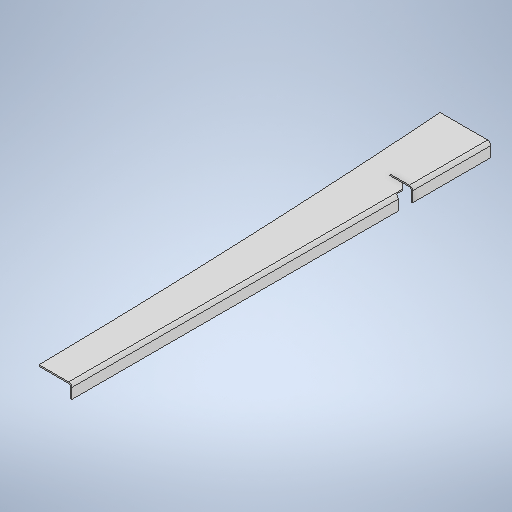
# Autodesk Inventor part: MSC 054 rib hip 1
Saved by Autodesk Inventor 2025 (Build 290162010, 162A)
## iProperties
Created: 2024-04-28
Part Number: MSC 054 rib hip 1
Material: Stainless Steel
Document SubType Name: Sheet Metal
Designer: pokla
Stock Number: МОО 054 шпангоут бедро 1
Density: 8 g/cm^3
Flat Pattern Width: 61.5 cm
Flat Pattern Length: 9.06945 cm
Flat Pattern Area: 557.771 cm^2
Sheet Metal Rule: AISI304 2mm Die16
Sheet Metal Width: 615,000 mm
Sheet Metal Length: 90,694 mm
Sheet Metal Area: 55777,098 mm^2
Appearance: Default
Стрингер_3: 66,766 mm
Стрингер_4: 48,009 mm
Стрингер_5: 51,895 mm
Стрингер_6: 78,448 mm
Author: admin
Autodesk Inventor part; units mm, degrees
ref_plane "YZ Plane" through (0, 0, 0) normal (1, 0, 0) x (0, 1, 0)
ref_plane "XZ Plane" through (0, 0, 0) normal (0, 1, 0) x (-1, 0, 0)
ref_plane "XY Plane" through (0, 0, 0) normal (0, 0, 1) x (1, 0, 0)
sketch "Sketch1" plane through (0, 0, 0) normal (0, 0, 1) x (1, 0, 0)
  arc A0 (750, -2100) -> (771.0671, -250.888) centre (-10250, -1050) ccw construction
  arc A1 (752.9864, -2100.2851) -> (772.2226, -225.7318) centre (-10246.9893, -1050.0309) ccw
  line L0 (-750, -2700) -> (-750, 0) construction
  line L1 (-800, 50) -> (-800, -2750) construction
  line L2 (-850, -2800) -> (-850, 100) construction
  line L3 (850, 100) -> (850, -2800)
  line L4 (800, -2750) -> (800, 50) construction
  line L5 (750, 0) -> (750, -2700) construction
  line L6 (771.0671, -250.888) -> (768.075, -251.105) construction
  line L7 (769.231, -225.9556) -> (772.2226, -225.7318) construction
  arc A2 (747.4657, -5.0326) -> (744.8748, -2.3426) centre (744.4792, -5.3164) ccw construction
  arc A3 (747.4657, -5.0326) -> (747.0136, -0.2851) centre (-10252.9897, -1050.251) ccw construction
  arc A4 (768.075, -251.105) -> (747.4657, -5.0326) centre (-10252.9897, -1050.251) ccw construction
  line L8 (750, 0) -> (747.0136, -0.2851) construction
  arc A5 (750.4522, -4.7486) -> (750, 0) centre (-10250, -1050) ccw construction
  arc A6 (750.4522, -4.7486) -> (745.2706, 0.6314) centre (744.4791, -5.3162) ccw
  line L9 (-750, 0) -> (750, 0) construction
  line L10 (-850, 100) -> (850, 100) construction
  line L11 (800, 50) -> (-800, 50) construction
  arc A7 (771.0671, -250.888) -> (750.4522, -4.7486) centre (-10250, -1050) ccw
  line L12 (750, -2700) -> (-750, -2700) construction
  line L13 (750, -2100) -> (752.9864, -2100.2851) construction
  line L14 (-800, -2750) -> (800, -2750)
  line L15 (850, -2800) -> (-850, -2800) construction
  arc A8 (110, -2700) -> (114.1118, -2698.3696) centre (110, -2694) ccw construction
  line L16 (0, -2697) -> (110, -2697) construction
  line L17 (0, -2700) -> (0, -2697) construction
  arc A9 (750, 0) -> (745.2706, 0.6314) centre (0, -5600) ccw construction
  line L18 (750, 0) -> (749.6018, -2.9735) construction
  arc A10 (750, -3.0268) -> (0, 47) centre (-0.2, -5603) ccw construction
  line L19 (0, 47) -> (0, 0) construction
  line L20 (0, 50) -> (0, 47) construction
  line L21 (0, 100) -> (0, 50)
  arc A11 (745.2706, 0.6314) -> (0, 50) centre (0, -5600) ccw construction
  line L22 (-750, -2100) -> (750, -2100) construction
  arc A12 (110, -2697) -> (112.0559, -2696.1848) centre (110, -2694) ccw construction
  line L23 (676.3163, -2173.4556) -> (674.2605, -2171.2708) construction
  line L24 (690.4112, -2151.9536) -> (692.4671, -2154.1384) construction
  line L25 (752.0559, -2102.1848) -> (676.3163, -2173.4556) construction
  line L26 (114.1118, -2698.3696) -> (750, -2100) construction
  arc A13 (752.0559, -2102.1848) -> (752.9864, -2100.2851) centre (749.9998, -2099.9999) ccw construction
  line L27 (750, -2100) -> (752.0559, -2102.1848) construction
  arc A14 (749.1768, -2100.7746) -> (750.1074, -2098.8746) centre (747.1209, -2098.5898) ccw construction
  line L28 (112.0559, -2696.1848) -> (690.4112, -2151.9536) construction
  line L29 (850, -270.888) -> (775.5075, -270.888)
  arc A15 (800, 50) -> (0, 100) centre (0, -6325) ccw construction
  arc A16 (825.5075, -270.888) -> (800, 50) centre (-10637.5382, -1020.6324) ccw construction
  line L30 (825.5075, -270.888) -> (825.5075, 100) construction
  arc A17 (790.2374, -2130.793) -> (825.5075, -270.888) centre (-10200.9329, -992.0761) ccw construction
  line L31 (0, -2700) -> (0, -2750) construction
  line L32 (112.3791, -2700) -> (132.2053, -2750) construction
  line L33 (132.2053, -2750) -> (850, -2074.5565)
  arc A18 (771.0107, -250.8921) -> (767.3384, -201.0273) centre (769.231, -225.9556) ccw construction
  line L34 (850, -400) -> (783.8747, -400) construction
  line L35 (850, -900) -> (801.9921, -900) construction
  line L36 (850, -1400) -> (797.4673, -1400) construction
  line L37 (850, -1900) -> (770.2723, -1900) construction
  line L38 (350, 100) -> (350, 39.1489)
  line L39 (-1472.612, -150) -> (-973.4947, -150)
  line L40 (-1472.612, -700) -> (-973.4947, -700)
  line L41 (-1472.612, -1250) -> (-973.4947, -1250)
  line L42 (-1472.612, -1800) -> (-973.4947, -1800)
  line L43 (800, -2750) -> (850, -2750) construction
  line L44 (752.9864, -2100.2851) -> (850, -2100.2851)
  point P0 (822.6583, -2100.2851)
  dimension "d16" = 1500
  dimension "d17" = 2700
  dimension "d18" = 2100
  dimension "d19" = 6
  dimension "d20" = 3
  dimension "d21" = 3
  dimension "d22" = 6
  dimension "d23" = 3
  dimension "d24" = 251.771
  dimension "d25" = 50
  dimension "d26" = 50
  dimension "d27" = 3
  dimension "d28" = 110
  dimension "d29" = 25
  dimension "d30" = 104
  dimension "d31" = 25
  dimension "d32" = 20
  dimension "d33" = 50
  dimension "d57" = 500
  dimension "d58" = 500
  dimension "d59" = 500
  dimension "d60" = 500
  dimension "d61" = 500
  dimension "d83" = 250
  dimension "d86" = 550
  dimension "d91" = 274.5565
  measures "d16" distance of L0.end L5.start
  measures "d17" distance of L5.start L5.end
  measures "d18" distance between parallel lines of L22 L9
  measures "d19" radius of A6
  measures "d20" radius of A2
  measures "d21" radius of A14
  measures "d22" radius of A8
  measures "d23" radius of A12
  measures "d24" distance of L6.start L5.start
  measures "d25" distance between parallel lines of L11 L10
  measures "d26" distance between parallel lines of L9 L11
  measures "d27" distance of L21.end L19.start
  measures "d28" distance from line of L17 A8.centre
  measures "d29" distance of L23.end L24.end
  measures "d30" distance of L27.start L23.end
  measures "d31" distance of L6.start L7.start
  measures "d32" vertical distance of L6.start L29.end
  measures "d33" distance of L30.start L29.end
  measures "d57" distance between parallel lines of L34 L10
  measures "d58" distance between parallel lines of L35 L34
  measures "d59" distance between parallel lines of L35 L36
  measures "d60" distance between parallel lines of L36 L37
  measures "d83" distance between parallel lines of L39 L10
  measures "d86" distance of L39.start L40.start
  measures "d91" distance from line of L33.end L42
extrude "Plate3" add sketch "Sketch1" along normal blind 2
sketch "Sketch3" plane through (848, -270.888, 2) normal (1, 0, 0) x (0, 1, 0)
  line L0 (-1829.397, 0) -> (0, 0)
  line L1 (0, 0) -> (0, 20)
  line L2 (0, 20) -> (-1829.397, 20)
  line L3 (-1829.397, 20) -> (-1829.397, 0)
  constraints: 6 end point, 1 horizontal, 1 perpendicular, 1 vertical
edge flange "Flange2" height 20 angle 90 thickness 2 bend radius 2.75 thickness toward (1, 0, 0) relief round relief width 2 relief depth 1 edges at (850, -1172.7223, 2) wall of the first edge with corners at (848, -2100.2851, 2) (848, -270.888, 2) (848, -270.888, -18) (848, -2100.2851, -18)
bend "Bend2"
corner "Corner2"
sketch "Sketch5" plane through (0, 0, 0) normal (0, 0, 1) x (1, 0, 0)
  line L0 (845.25, -2100.2851) -> (845.25, -270.888) projected
  line L1 (775.5075, -270.888) -> (845.25, -270.888) projected
  arc A0 (752.9864, -2100.2851) -> (775.5075, -270.888) centre (-10246.9893, -1050.0309) ccw projected
  line L2 (850, -270.888) -> (850, -2100.2851) projected
  line L3 (850, -385.888) -> (818, -385.888)
  line L4 (850, -387.888) -> (848, -387.888) construction
  line L5 (848, -2100.2851) -> (848, -270.888) projected
  line L6 (818, -385.888) -> (818, -387.888)
  line L7 (850, -885.887) -> (801.7915, -885.887) construction
  line L8 (850, -887.887) -> (801.821, -887.887) construction
  line L9 (819, -885.887) -> (819, -887.887) construction
  line L10 (850, -1385.887) -> (797.9055, -1385.887) construction
  line L11 (850, -1387.887) -> (797.8445, -1387.887) construction
  line L12 (819, -1385.887) -> (819, -1387.887) construction
  line L13 (850, -1885.887) -> (771.352, -1885.887) construction
  line L14 (850, -1887.887) -> (771.2001, -1887.887) construction
  line L15 (819, -1885.887) -> (819, -1887.887) construction
  line L16 (850, -906.887) -> (845.25, -906.887) construction
  line L17 (845.25, -1406.887) -> (850, -1406.887) construction
  line L18 (845.25, -1906.887) -> (850, -1906.887) construction
  line L19 (845.25, -2100.2851) -> (752.9864, -2100.2851) projected
  line L20 (850, -385.888) -> (850, -406.888)
  line L21 (848, -385.888) -> (848, -387.888) construction
  line L22 (850, -406.888) -> (848, -406.888)
  line L23 (818, -385.888) -> (783.034, -385.888) construction
  line L24 (818, -387.888) -> (783.1542, -387.888) construction
  line L25 (848, -387.888) -> (848, -406.888)
  line L26 (848, -387.888) -> (818, -387.888)
  line L27 (848, -406.888) -> (845.25, -406.888)
  point P0 (0, 0)
  point P1 (845.25, -380.4205)
  point P2 (848, -380.4205)
  point P3 (848, -1906.887)
  point P4 (848, -1887.887)
  point P5 (848, -1406.887)
  point P6 (848, -1387.887)
  point P7 (848, -906.887)
  point P8 (848, -887.887)
  point P9 (818, -386.888)
  point P10 (848, -406.888)
  point P11 (850, -410.4205)
  point P12 (848, -385.888)
  point P13 (819, -886.887)
  point P14 (819, -1386.887)
  point P15 (819, -1886.887)
  point P16 (848, -406.888)
  point P17 (845.25, -387.888)
  dimension "d69" = 1829.397
  dimension "d70" = 2
  dimension "d76" = 66.966
  dimension "d80" = 48.2085
  dimension "d81" = 31
  dimension "d94" = 21
  dimension "d95" = 31
  dimension "d96" = 21
  dimension "d97" = 31
  dimension "d98" = 21
  dimension "d102" = 78.648
  dimension "d104" = 52.0945
  dimension "d106" = 2
  dimension "d107" = 21
  dimension "d108" = 116
  dimension "d109" = 500
  dimension "d110" = 500
  dimension "d111" = 500
  dimension "d112" = 32
  constraints: 46 end point, 14 perpendicular, 13 point on line, 7 horizontal, 4 midpoint, 3 equal length, 3 parallel, 2 vertical, 22 other
  measures "d69" distance of point (850, -270.888) point (850, -2100.285)
  measures "d70" distance between parallel lines of L4 L3
  measures "d76" distance of L3.start L23.end
  measures "d80" distance of L7.start L7.end
  measures "d94" distance of L16.start L7.start
  measures "d95" distance of L12.start L10.start
  measures "d96" distance of L17.end L10.start
  measures "d97" distance of L15.start L13.start
  measures "d98" distance of L18.end L13.start
  measures "d102" distance of L13.start L13.end
  measures "d104" distance of L10.end L10.start
  measures "d106" distance of L22.end L20.end
  measures "d107" distance of L20.end L3.start
  measures "d108" vertical distance of point (850, -270.888) point (818, -386.888)
  measures "d109" distance of point (819, -886.887) point (818, -386.888)
  measures "d110" distance of point (819, -1386.887) point (819, -886.887)
  measures "d111" distance of point (819, -1886.887) point (819, -1386.887)
  measures "d112" distance of L3.end L3.start
extrude "Extrusion2" cut sketch "Sketch5" along normal through all both and the other way through all contours L0 L26 L5 L27 | L26 L6 L3 L0 | L0 L3 L5 L26 | L5 L3 L2 L22
chamfer "Chamfer2" distance 8 angle 45 1 edges at (845.25, -387.888, 1)
pattern_linear "Rectangular Pattern3" count 4 spacing 500 along (0, -1, 0) of "Extrusion2", "Chamfer2"
sketch "Sketch6" plane through (0, 0, 0) normal (0, 0, -1) x (-1, 0, 0)
  line L0 (-803.1643, -805.888) -> (-817.1643, -805.888) construction
  line L1 (-817.1643, -805.888) -> (-817.1643, -605.888) construction
  line L2 (-817.1643, -605.888) -> (-803.1643, -605.888) construction
  line L3 (-803.1643, -605.888) -> (-803.1643, -805.888) construction
  line L4 (-752.9864, -2100.2851) -> (-845.25, -2100.2851) projected
  line L5 (-803.1643, -1810.888) -> (-803.1643, -1860.888) construction
  line L6 (-803.1643, -1860.888) -> (-815.1643, -1860.888) construction
  line L7 (-815.1643, -1860.888) -> (-815.1643, -1810.888) construction
  line L8 (-815.1643, -1810.888) -> (-803.1643, -1810.888) construction
  line L9 (-845.25, -1885.888) -> (-818, -1885.888) projected
  line L10 (-803.1643, -1310.888) -> (-803.1643, -1360.888) construction
  line L11 (-803.1643, -1360.888) -> (-815.1643, -1360.888) construction
  line L12 (-815.1643, -1360.888) -> (-815.1643, -1310.888) construction
  line L13 (-815.1643, -1310.888) -> (-803.1643, -1310.888) construction
  line L14 (-803.1643, -810.888) -> (-803.1643, -860.888) construction
  line L15 (-803.1643, -860.888) -> (-815.1643, -860.888) construction
  line L16 (-815.1643, -860.888) -> (-815.1643, -810.888) construction
  line L17 (-815.1643, -810.888) -> (-803.1643, -810.888) construction
  line L18 (-803.1643, -310.888) -> (-803.1643, -360.888) construction
  line L19 (-803.1643, -360.888) -> (-815.1643, -360.888) construction
  line L20 (-815.1643, -360.888) -> (-815.1643, -310.888) construction
  line L21 (-815.1643, -310.888) -> (-803.1643, -310.888) construction
  line L22 (-845.25, -1385.888) -> (-818, -1385.888) projected
  line L23 (-845.25, -885.888) -> (-818, -885.888) projected
  line L24 (-845.25, -385.888) -> (-818, -385.888) projected
  point P0 (0, 0)
  point P1 (-753.1643, -2098.4205)
  point P2 (-824.6397, -2098.4205)
  dimension "d120" = 200
  dimension "d121" = 14
  dimension "d124" = 50
  dimension "d125" = 12
  dimension "d126" = 50
  dimension "d127" = 25
  dimension "d128" = 50
  dimension "d129" = 12
  dimension "d130" = 50
  dimension "d131" = 12
  dimension "d132" = 50
  dimension "d133" = 12
  dimension "d134" = 50
  dimension "d135" = 25
  dimension "d136" = 25
  dimension "d137" = 25
  dimension "d138" = 50
  dimension "d139" = 50
  dimension "d140" = 50
  dimension "d143" = 80
  constraints: 11 other
  measures "d120" distance of L0.end L1.end
  measures "d121" distance of L1.end L2.end
  measures "d124" horizontal distance of point (-753.164, -2098.421) L0.start
  measures "d125" distance of L7.end L5.start
  measures "d126" distance of L6.end L7.end
  measures "d127" distance between parallel lines of L9 L6
  measures "d128" horizontal distance of point (-753.164, -2098.421) L5.end
  measures "d129" distance of L13.start L13.end
  measures "d130" distance of L11.end L13.start
  measures "d131" distance of L17.start L17.end
  measures "d132" distance of L15.end L17.start
  measures "d133" distance of L21.start L21.end
  measures "d134" distance of L19.end L21.start
  measures "d135" distance between parallel lines of L22 L11
  measures "d136" distance between parallel lines of L23 L15
  measures "d137" distance between parallel lines of L24 L19
  measures "d138" horizontal distance of point (-753.164, -2098.421) L10.end
  measures "d139" horizontal distance of point (-753.164, -2098.421) L14.end
  measures "d140" horizontal distance of point (-753.164, -2098.421) L18.end
  measures "d143" distance between parallel lines of L0 L23
mark "Mark1"
sketch "Sketch7" plane through (0, 0, 0) normal (0, 0, 1) x (1, 0, 0)
  line L0 (837.25, -1887.888) -> (845.25, -1895.888) construction
  line L1 (837.25, -1887.888) -> (818, -1887.888) construction
  line L2 (818, -1887.888) -> (818, -1885.888) construction
  line L3 (818, -1885.888) -> (845.25, -1885.888) construction
  line L4 (845.25, -1885.888) -> (845.25, -1406.888) construction
  line L5 (845.25, -1406.888) -> (845.25, -1395.888) construction
  line L6 (837.25, -1387.888) -> (845.25, -1395.888) construction
  line L7 (837.25, -1387.888) -> (818, -1387.888) construction
  line L8 (818, -1387.888) -> (818, -1385.888) construction
  line L9 (818, -1385.888) -> (845.25, -1385.888) construction
  line L10 (845.25, -1385.888) -> (845.25, -906.888) construction
  line L11 (845.25, -906.888) -> (845.25, -895.888) construction
  line L12 (837.25, -887.888) -> (845.25, -895.888) construction
  line L13 (837.25, -887.888) -> (818, -887.888) construction
  line L14 (818, -887.888) -> (818, -885.888) construction
  line L15 (818, -885.888) -> (845.25, -885.888) construction
  line L16 (845.25, -885.888) -> (845.25, -406.888) construction
  line L17 (845.25, -406.888) -> (845.25, -395.888) projected
  line L18 (837.25, -387.888) -> (845.25, -395.888) projected
  line L19 (837.25, -387.888) -> (818, -387.888) projected
  line L20 (818, -387.888) -> (818, -385.888) projected
  line L21 (818, -385.888) -> (845.25, -385.888) projected
  line L22 (845.25, -385.888) -> (845.25, -270.888) projected
  line L23 (775.5075, -270.888) -> (845.25, -270.888) projected
  arc A0 (752.9864, -2100.2851) -> (775.5075, -270.888) centre (-10246.9893, -1050.0309) ccw construction
  line L24 (845.25, -2100.2851) -> (752.9864, -2100.2851) construction
  line L25 (845.25, -2100.2851) -> (845.25, -1906.888) construction
  line L26 (845.25, -1906.888) -> (845.25, -1895.888) construction
  line L27 (716.6808, -2324.332) -> (990.5996, -2324.332)
  line L28 (990.5996, -2324.332) -> (990.5996, -885.888)
  line L29 (990.5996, -885.888) -> (716.6808, -885.888)
  line L30 (716.6808, -885.888) -> (716.6808, -2324.332)
  line L31 (848, -1385.888) -> (845.25, -1385.888) projected
  line L32 (845.25, -906.888) -> (845.25, -1385.888) projected
  line L33 (845.25, -906.888) -> (848, -906.888) projected
  line L34 (848, -1385.888) -> (848, -906.888) projected
  line L35 (848, -885.888) -> (845.25, -885.888) projected
  line L36 (845.25, -406.888) -> (845.25, -885.888) projected
  line L37 (845.25, -406.888) -> (848, -406.888) projected
  line L38 (848, -885.888) -> (848, -406.888) projected
  point P0 (0, 0)
  constraints: 8 end point, 2 parallel, 1 horizontal, 1 perpendicular, 1 point on line
extrude "Extrusion3" cut sketch "Sketch7" along normal through all both and the other way through all contours L30 L29 L28 L27 | L31 L32 L33 L34
equation "\"d16\" = d34"
equation "\"d17\" = d35"
equation "\"d18\" = d36"
equation "\"d19\" = d37"
equation "\"d20\" = d38"
equation "\"d21\" = d39"
equation "\"d22\" = d39 + d43"
equation "\"d23\" = d39"
equation "\"d27\" = d39"
equation "\"d28\" = 0.5 * d44"
equation "\"d29\" = d41"
equation "\"d30\" = d42"
equation "\"d31\" = d41"
equation "\"d33\" = d25"
equation "\"Стрингер_3\" = 66.766"
equation "\"d37\" = d39 + d43"
equation "\"d38\" = d39"
equation "\"d43\" = d39"
equation "\"Стрингер_4\" = 48.00853"
equation "\"Стрингер_5\" = 51.89453"
equation "\"Стрингер_6\" = 78.44803"
equation "\"d34\" = 1500"
equation "\"d35\" = 2700"
equation "\"d36\" = 2100"
equation "\"d39\" = 3"
equation "\"d44\" = 220"
equation "\"d41\" = 25"
equation "\"d42\" = 104"
body "Solid2"
